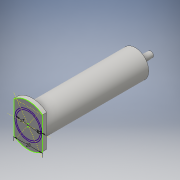
# Autodesk Inventor part: Small Syringe
Saved by Autodesk Inventor 2016 (Build 200138000, 138)
## iProperties
Created: 2016-05-08
Part Number: Small Syringe
Material: Generic
Document SubType Name: Modeling
Designer: Kenneth Daniel
Density: 1 g/cm^3
Appearance: Default
Author: Kenneth Daniel
Autodesk Inventor part; units mm, degrees
ref_plane "YZ Plane" through (0, 0, 0) normal (1, 0, 0) x (0, 1, 0)
ref_plane "XZ Plane" through (0, 0, 0) normal (0, 1, 0) x (-1, 0, 0)
ref_plane "XY Plane" through (0, 0, 0) normal (0, 0, 1) x (1, 0, 0)
sketch "Sketch1" plane through (0, 0, 0) normal (0, 1, 0) x (-1, 0, 0)
  circle A0 centre (0, 0) radius 8.5
  line L0 (10, -11.1988) -> (10, 11.1988)
  line L1 (-10, 11.1988) -> (-10, -11.1988)
  line L2 (-10, -14.792) -> (10, 14.792) construction
  line L3 (10, -14.792) -> (-10, 14.792) construction
  line L4 (10, 11.1988) -> (-10, 11.1988) construction
  arc A1 (10, 11.1988) -> (-10, 11.1988) centre (0, -0.9197) ccw
  line L5 (14.8819, 0) -> (-15.6848, 0) construction
  arc A2 (-10, -11.1988) -> (10, -11.1988) centre (0, 0.9197) ccw
  circle A3 centre (0, 0) radius 9.5
  dimension "d0" = 17
  dimension "d1" = 20
  dimension "d2" = 1
  constraints: 12 end point, 4 centre point, 4 point on circle, 3 symmetric about line, 2 midpoint, 1 coincident, 1 horizontal, 1 parallel, 1 perpendicular, 1 other
  measures "d0" diameter of A0
  measures "d1" distance of L2.start L3.start
  measures "d2" radial gap between concentric circles of A0 A3
extrude "Extrusion1" add sketch "Sketch1" along normal blind 75 contours A3
extrude "Extrusion2" add sketch "Sketch1" along normal blind 3
sketch "Sketch2" plane through (0, 0, 0) normal (0, 0, 1) x (1, 0, 0)
  line L0 (9.5, 75) -> (-9.5, 75) projected
  line L1 (-9.5, 75) -> (-7.5, 75)
  line L2 (-7.5, 75) -> (-3.4008, 77.3135)
  line L3 (-3.4008, 77.3135) -> (-2.4311, 78.5256)
  line L4 (-2.4311, 78.5256) -> (-1.9463, 85.879)
  line L5 (-1.9463, 85.879) -> (-0.9463, 85.879)
  line L6 (-0.9463, 85.879) -> (-0.9463, 78.5256)
  line L7 (-0.9463, 78.5256) -> (-3.4008, 75)
  line L8 (-3.4008, 75) -> (-9.5, 75)
  line L9 (-3.4008, 77.3135) -> (-9.5, 75)
  line L10 (0, -17.1758) -> (0, 103.0548) projected
  point P0 (0, 0)
  dimension "d7" = 2
  dimension "d8" = 1
  constraints: 18 end point, 2 point on line, 1 collinear, 1 horizontal, 1 perpendicular
  measures "d7" distance of L0.end L1.end
  measures "d8" distance of L4.end L5.end
revolve "Revolution1" add sketch "Sketch2" angle 360 about axis through (0, -10, 0) along (0, 1, 0)
body "Solid1"
